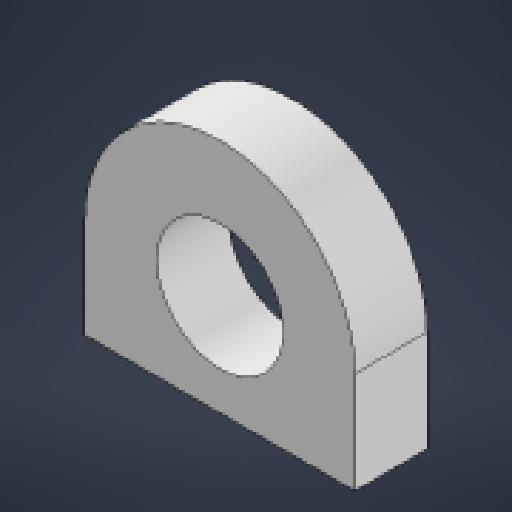
# Autodesk Inventor part: 3DPRINT,VERTICAL,ROLLER,TOP,BEARING,BLOCK
Saved by Autodesk Inventor 2026 (Build 300175000, 175)
## iProperties
Created: 2026-03-31
Part Number: 3DPRINT,VERTICAL,ROLLER,TOP,BEARING,BLOCK
Material: Generic
Document SubType Name: Modeling
Designer: littl
Density: 1 g/cm^3
Appearance: Default
Author: littl
Autodesk Inventor part; units mm, degrees
ref_plane "YZ Plane" through (0, 0, 0) normal (1, 0, 0) x (0, 1, 0)
ref_plane "XZ Plane" through (0, 0, 0) normal (0, 1, 0) x (-1, 0, 0)
ref_plane "XY Plane" through (0, 0, 0) normal (0, 0, 1) x (1, 0, 0)
sketch "Sketch1" plane through (0, 0, 0) normal (0, 0, 1) x (1, 0, 0)
  circle A0 centre (0, 0) radius 11.1125
  arc A1 (20.6375, 0) -> (-20.6375, 0) centre (0, 0) ccw
  line L0 (20.6375, 0) -> (20.6375, -17.907)
  line L1 (20.6375, -17.907) -> (-20.6375, -17.907)
  line L2 (-20.6375, -17.907) -> (-20.6375, 0)
  dimension "d0" = 22.225
  dimension "d2" = 9.525
  dimension "d3" = 17.907
  constraints: 6 end point, 2 centre point, 2 coincident, 2 perpendicular, 2 point on circle, 2 tangent, 1 vertical
  measures "d0" diameter of A0
  measures "d2" radial gap between concentric circles of A0 A1
  measures "d3" distance from line of point (0, 0) L1
extrude "Extrusion1" add sketch "Sketch1" along normal blind 9.525
sketch "Sketch2" plane through (-20.6375, -17.907, 0) normal (0, -1, 0) x (1, 0, 0)
  circle A0 centre (6.35, 4.7625) radius 2.8195
  circle A1 centre (34.925, 4.7625) radius 2.8195
  line L0 (0, 0) -> (0, 9.525) projected
  line L1 (41.275, 0) -> (41.275, 9.525) projected
  point P0 (20.6375, 0)
  point P1 (0, 4.7625)
  point P2 (41.275, 4.7625)
  dimension "d6" = 5.639
  dimension "d7" = 6.35
  dimension "d8" = 6.35
  constraints: 2 centre point, 2 coincident, 2 horizontal alignment, 2 midpoint, 1 equal radius
  measures "d6" diameter of A0
  measures "d7" distance from line of L0 A0.centre
  measures "d8" distance from line of L1 A1.centre
hole "Hole1" at (-14.2875, -17.907, 4.7625) at (14.2875, -17.907, 4.7625) direction (0, 1, 0) diameter 3.9624 depth 13.6144 tip angle 118 thread size "10-32 UNF" class "2B" standard "ANSI Unified Screw Threads"
body "Solid1"
